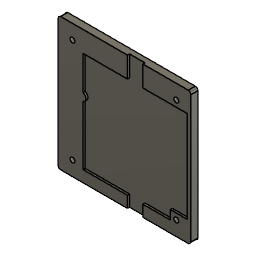
AlignerAL (Autodesk Fusion 360 design; units mm, degrees)
part number: 2026-08-13-12-31-00-775
Autodesk Fusion 360 part; units mm, degrees
ref_plane "WorkPlane1" through (0, 0, 7) normal (0, 0, 1) x (1, 0, 0)
sketch "Square Base Plate Sketch" plane through (0, 0, 0) normal (0, 0, 1) x (1, 0, 0)
  line L0 (-65, -65) -> (65, -65)
  line L1 (65, -65) -> (65, 65)
  line L2 (65, 65) -> (-65, 65)
  line L3 (-65, 65) -> (-65, -65)
extrude "Square Base Plate" add sketch "Square Base Plate Sketch" along normal blind 7
fillet "Fillet1" radius 2.5 4 edges at (-65, 65, 3.5) (65, 65, 3.5) (65, -65, 3.5) (-65, -65, 3.5)
sketch "Wafer Nest Pocket Sketch" plane through (0, 0, 7) normal (0, 0, 1) x (1, 0, 0)
  line L0 (-40.523, -53.7567) -> (61.477, -53.7567)
  line L1 (61.477, -53.7567) -> (61.477, 44.704)
  line L2 (61.477, 44.704) -> (-40.523, 44.704)
  line L3 (-40.523, 44.704) -> (-40.523, -53.7567)
extrude "Wafer Nest Pocket" cut sketch "Wafer Nest Pocket Sketch" against normal blind 2
sketch "Front-Center Access Relief Sketch" plane through (0, 0, 7) normal (0, 0, 1) x (1, 0, 0)
  line L0 (2.977, -66) -> (17.977, -66)
  line L1 (17.977, -66) -> (17.977, -50.7567)
  line L2 (17.977, -50.7567) -> (2.977, -50.7567)
  line L3 (2.977, -50.7567) -> (2.977, -66)
extrude "Front-Center Access Relief" cut sketch "Front-Center Access Relief Sketch" against normal blind 2
sketch "Rear-Center Access Relief Sketch" plane through (0, 0, 7) normal (0, 0, 1) x (1, 0, 0)
  line L0 (2.977, 41.704) -> (17.977, 41.704)
  line L1 (17.977, 41.704) -> (17.977, 66)
  line L2 (17.977, 66) -> (2.977, 66)
  line L3 (2.977, 66) -> (2.977, 41.704)
extrude "Rear-Center Access Relief" cut sketch "Rear-Center Access Relief Sketch" against normal blind 2
sketch "X Datum Bump Sketch (165 deg / 9:30)" plane through (0, 0, 7) normal (0, 0, 1) x (1, 0, 0)
  circle A0 centre (-41.683, 7.6802) radius 4
extrude "X Datum Bump (165 deg / 9:30)" add sketch "X Datum Bump Sketch (165 deg / 9:30)" against normal blind 2
sketch "Front-Right Corner Clip (dowel) Sketch" plane through (0, 0, 7) normal (0, 0, 1) x (1, 0, 0)
  line L0 (44.9187, -53.7567) -> (61.477, -53.7567)
  line L1 (61.477, -53.7567) -> (61.477, -44.9187)
  line L2 (61.477, -44.9187) -> (44.9187, -44.9187)
  line L3 (44.9187, -44.9187) -> (44.9187, -53.7567)
extrude "Front-Right Corner Clip (dowel)" add sketch "Front-Right Corner Clip (dowel) Sketch" against normal blind 2
sketch "Outer Front Left Dowel Bore Sketch" plane through (0, 0, 7) normal (0, 0, 1) x (1, 0, 0)
  circle A0 centre (-50.8, -50.8) radius 2.3813
extrude "Outer Front Left Dowel Bore" cut sketch "Outer Front Left Dowel Bore Sketch" against normal blind 7
sketch "Outer Front Right Dowel Bore Sketch" plane through (0, 0, 7) normal (0, 0, 1) x (1, 0, 0)
  circle A0 centre (50.8, -50.8) radius 2.3813
extrude "Outer Front Right Dowel Bore" cut sketch "Outer Front Right Dowel Bore Sketch" against normal blind 7
sketch "Outer Rear Left Dowel Bore Sketch" plane through (0, 0, 7) normal (0, 0, 1) x (1, 0, 0)
  circle A0 centre (-50.8, 50.8) radius 2.3813
extrude "Outer Rear Left Dowel Bore" cut sketch "Outer Rear Left Dowel Bore Sketch" against normal blind 7
sketch "Outer Rear Right Dowel Bore Sketch" plane through (0, 0, 7) normal (0, 0, 1) x (1, 0, 0)
  circle A0 centre (50.8, 50.8) radius 2.3813
extrude "Outer Rear Right Dowel Bore" cut sketch "Outer Rear Right Dowel Bore Sketch" against normal blind 7
equation "gridPitch = 25.4 mm" comment "Table hole-grid pitch"
equation "indexMove = 50.8 mm" comment "Two-grid-space indexing move"
equation "outerPinPatternSpan = 101.6 mm" comment "Four-space outer pin span"
equation "dowelDiameter = 4.7625 mm" comment "3/16 in steel locating dowel diameter"
equation "dowelHoleDiameter = 4.7625 mm" comment "3/16 in reamed dowel bore"
equation "basePlateSize = 130.0 mm" comment "Square base plate side length"
equation "baseThickness = 7.0 mm" comment "Base plate thickness"
equation "pocketDepth = 2.0 mm" comment "Wafer-nest pocket depth"
equation "nestClearance = 1.0 mm" comment "Loose gap at left/right/rear pocket walls"
equation "filletRadius = 2.5 mm" comment "Base-plate corner fillet radius"
equation "primaryFlatClearance = 0.175 mm" comment "Front wall forward of nominal flat"
equation "xBumpDiameter = 8.0 mm" comment "X-datum bump diameter"
equation "nestReliefWidth = 15.0 mm" comment "Front/rear access relief width"
equation "nestOffsetX = 7.29 mm" comment "Nest X from pin-square center"
equation "nestOffsetY = -4.95 mm" comment "Nest Y from pin-square center"
